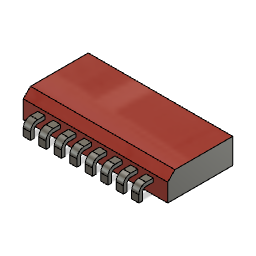
Multiplexer (8-8) v1 (Autodesk Fusion 360 design; units mm, degrees)
Autodesk Fusion 360 part; units mm, degrees
sketch "Sketch1" plane through (0, 0, 0) normal (0, 1, 0) x (1, 0, 0)
  line L0 (0, 0) -> (20, 0)
  line L1 (20, 0) -> (20, 9)
  line L2 (20, 9) -> (0, 9)
  line L3 (0, 9) -> (0, 0)
  dimension "d1" = 20
  dimension "d2" = 9
  constraint horizontal L0
  constraint vertical L1
  constraint horizontal L2
  constraint vertical L3
  constraint coincident L0.start L3.end
  measures "d1" distance of L0.start L0.end
  measures "d2" distance of L0.end L1.end
extrude "Extrude1" add sketch "Sketch1" along normal mid plane 3.5 makes body 1
chamfer "Chamfer1" distance 1 angle 45 1 edges at (10, 1.75, 0) on bodies 1
sketch "Sketch2" plane through (0, 0, 0) normal (0, 1, 0) x (1, 0, 0)
  line L0 (2, -2) -> (3, -2)
  line L1 (3, -2) -> (3, 11)
  line L2 (3, 11) -> (2, 11)
  line L3 (2, 11) -> (2, -2)
  line L4 (20, 0) -> (0, 0)
  dimension "d6" = 1
  dimension "d7" = 13
  dimension "d8" = 2
  dimension "d9" = 2
  constraint horizontal L0
  constraint vertical L1
  constraint horizontal L2
  constraint vertical L3
  measures "d6" distance of L0.start L0.end
  measures "d7" distance of L0.end L1.end
  measures "d8" distance of L0 L4
  measures "d9" distance of L4.end L3
extrude "Extrude2" add sketch "Sketch2" along normal mid plane 0.5 separate body makes body 2
sketch "Sketch3" plane through (0, 0, 2) normal (0, 0, 1) x (1, 0, 0)
  line L0 (3, -0.25) -> (3, 0.25)
  line L1 (3, 0.25) -> (2, 0.25)
  line L2 (2, 0.25) -> (2, -0.25)
  line L3 (2, -0.25) -> (3, -0.25)
  line L4 (2, 0.25) -> (3, 0.25)
  line L5 (3, 0.25) -> (3, -1.75)
  line L6 (3, -1.75) -> (2, -1.75)
  line L7 (2, -1.75) -> (2, 0.25)
  dimension "d14" = 2
  constraint horizontal L4
  constraint vertical L5
  constraint horizontal L6
  constraint vertical L7
  constraint coincident L1.end L2.start
  measures "d14" distance of L1.end L6.end
extrude "Extrude3" add sketch "Sketch3" against normal blind 0.5 contours L3 L5 L6 L7 bodies 2
fillet "Fillet1" radius 1 1 edges at (2.5, 0.25, 2) on bodies 2
fillet "Fillet2" radius 0.5 1 edges at (2.5, -0.25, 1.5) on bodies 2
sketch "Sketch4" plane through (0, 0, -11) normal (0, 0, -1) x (-1, 0, 0)
  line L0 (-2, -0.25) -> (-2, 0.25)
  line L1 (-2, 0.25) -> (-3, 0.25)
  line L2 (-3, 0.25) -> (-3, -0.25)
  line L3 (-3, -0.25) -> (-2, -0.25)
  line L4 (-3, 0.25) -> (-2, 0.25)
  line L5 (-2, 0.25) -> (-2, -1.75)
  line L6 (-2, -1.75) -> (-3, -1.75)
  line L7 (-3, -1.75) -> (-3, 0.25)
  dimension "d21" = 2
  constraint horizontal L4
  constraint vertical L5
  constraint horizontal L6
  constraint vertical L7
  constraint coincident L1.end L2.start
  measures "d21" distance of L1.end L6.end
extrude "Extrude4" add sketch "Sketch4" against normal blind 0.5 contours L3 L5 L6 L7 bodies 2
fillet "Fillet3" radius 1 1 edges at (2.5, 0.25, -11) on bodies 2
fillet "Fillet4" radius 0.5 1 edges at (2.5, -0.25, -10.5) on bodies 2
pattern_path "PathPattern2" count 8 spacing 2.1429 from (2.5, 0.75, 0) along 1 edges at (10, 0.75, 0) of bodies 2 on bodies 1 makes body 3 at (4.4762, -0.25, -6.3333) makes body 4 at (6.619, -0.25, -6.3333) makes body 5 at (8.7619, -0.25, -6.3333) makes body 6 at (10.9048, -0.25, -6.3333) makes body 7 at (13.0476, -0.25, -6.3333) makes body 8 at (15.1905, -0.25, -6.3333) makes body 9 at (17.3333, -0.25, -6.3333)
combine "Combine1" operation add target body 1 tool bodies 2 8 4 6 7 3 5 9
